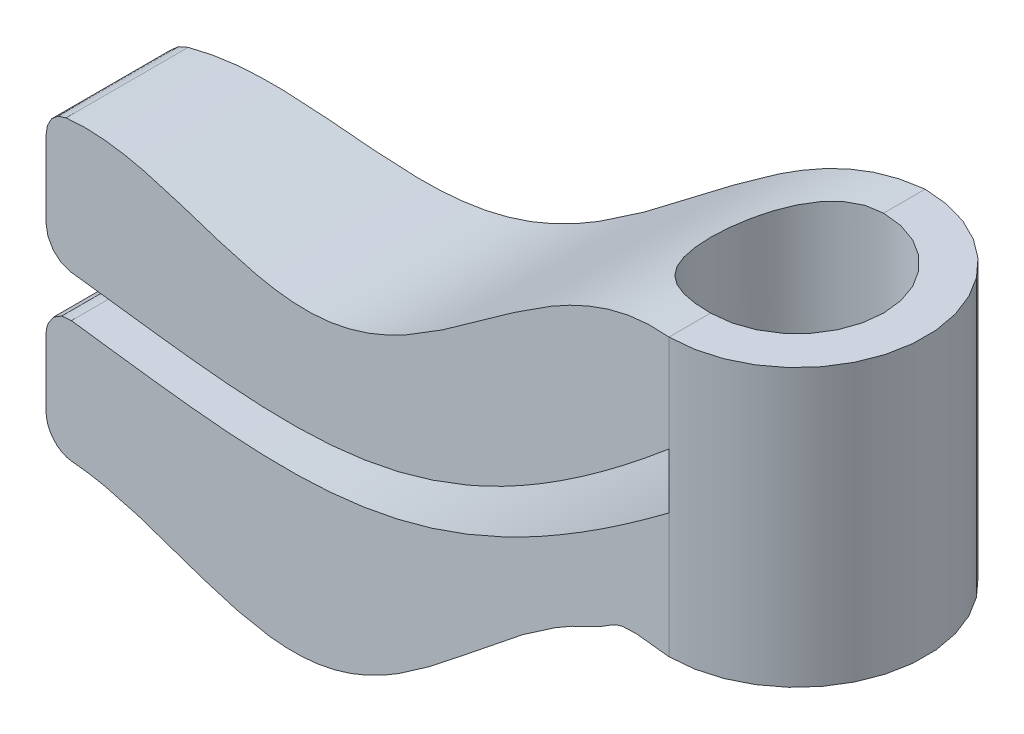
# Autodesk Inventor part: Fahne
Saved by Autodesk Inventor 2020 (Build 240168000, 168)
## iProperties
Created: 2020-05-10
Part Number: Fahne
Material: Generisch
Document SubType Name: Modeling
Designer: MartinDJay
Density: 1 g/cm^3
Appearance: Vorgabe
Author: MartinDJay
Autodesk Inventor part; units mm, degrees
ref_plane "YZ Plane" through (0, 0, 0) normal (1, 0, 0) x (0, 1, 0)
ref_plane "XZ Plane" through (0, 0, 0) normal (0, 1, 0) x (-1, 0, 0)
ref_plane "XY Plane" through (0, 0, 0) normal (0, 0, 1) x (1, 0, 0)
sketch "Skizze1" plane through (0, 0, 0) normal (0, 1, 0) x (-1, 0, 0)
  circle A0 centre (0, 0) radius 6.25
  circle A1 centre (0, 0) radius 9.25
  dimension "d0" = 12.5
  dimension "d2" = 3
  constraints: 2 centre point, 2 coincident
  measures "d0" diameter of A0
  measures "d2" radial gap between concentric circles of A1 A0
extrude "Extrusion1" add sketch "Skizze1" along normal blind 20
sketch "Skizze2" plane through (0, 20, 0) normal (0, 1, 0) x (1, 0, 0)
  circle A0 centre (0, 0) radius 9.25 projected
  line L0 (0, -9.25) -> (-50, -9.25)
  line L1 (-50, -9.25) -> (-50, 9.25)
  line L2 (-50, 9.25) -> (0, 9.25)
  line L3 (-50, 0) -> (0, 0) construction
  dimension "d5" = 50
  constraints: 8 end point, 2 horizontal, 2 point on circle, 2 tangent, 1 midpoint, 1 perpendicular, 1 point on line
  measures "d5" distance of L0.start L0.end
extrude "Extrusion2" add sketch "Skizze2" against normal blind 45 contours A0 L0 L1 L2
sketch "Skizze3" plane through (-50, 20, 9.25) normal (0, 0, 1) x (1, 0, 0)
  line L0 (0, 0) -> (0, -45) projected
  spline S0 degree 4 poles (50, -20) (33.6893, -20) (25.205, -49.5147) (14.9206, -32.0469) (0, -34.3156) knots 0 0 0 0 0 1 1 1 1 1
  line L1 (50, -20) -> (50, -45)
  line L2 (50, -45) -> (0, -45)
  line L3 (0, -45) -> (0, -34.3156)
  line L4 (59.25, -20) -> (50, -20) projected
  line L5 (50, -45) -> (0, -45) projected
  line L6 (50, -20) -> (50, 0) projected
  spline S1 degree 4 poles (50, 0) (34.1322, 0) (24.5091, -28.0895) (15.116, -8.5647) (0, -13.3156) knots 0 0 0 0 0 1 1 1 1 1
  line L7 (0, -13.3156) -> (0, 0)
  line L8 (0, 0) -> (50, 0) projected
  line L9 (59.25, 0) -> (50, 0) projected
  spline S2 degree 3 poles (50, -7) (29.5788, -24.5812) (20.0225, -22.4161) (0, -22.3156) knots 0 0 0 0 1 1 1 1
  spline S3 degree 3 poles (50, -11) (29.3142, -27.0201) (20.0053, -25.6187) (0, -25.3156) knots 0 0 0 0 1 1 1 1
  line L10 (0, -22.3156) -> (0, -25.3156)
  line L11 (50, -7) -> (50, -11)
  point P0 (30, -31.7804)
  point P1 (17, -36.3156)
  point P2 (30, -10.7804)
  point P3 (17, -14.3156)
  point P4 (30, -19.7804)
  point P5 (17, -22.3156)
  point P6 (30, -22.7804)
  point P7 (17, -25.3156)
  point P8 (0, -25.3156)
  dimension "d11" = 20
  dimension "d12" = 13
  dimension "d16" = 8
  dimension "d17" = 9
  dimension "d18" = 7
  dimension "d19" = 9
  dimension "d20" = 4
  dimension "d21" = 9
  dimension "d22" = 11
  dimension "d23" = 9
  dimension "d26" = 3
  dimension "d27" = 3
  dimension "d28" = 3
  constraints: 12 end point, 7 vertical alignment, 5 point on line, 2 horizontal, 2 perpendicular, 2 vertical, 1 collinear, 1 parallel, 16 other
  measures "d11" distance from line of L1 point (30, -31.78)
  measures "d12" horizontal distance of point (30, -31.78) point (17, -36.316)
  measures "d16" distance of point (17, -14.316) point (17, -22.316)
  measures "d17" distance of point (30, -10.78) point (30, -19.78)
  measures "d18" distance of L6.end L11.start
  measures "d19" distance of L7.start L10.start
  measures "d20" distance of L11.start L11.end
  measures "d21" distance of point (30, -22.78) point (30, -31.78)
  measures "d22" distance of point (17, -36.316) point (17, -25.316)
  measures "d23" distance of L3.end L10.end
  measures "d26" distance of point (30, -22.78) point (30, -19.78)
  measures "d27" distance of point (17, -22.316) point (17, -25.316)
  measures "d28" distance of L10.start L10.end
extrude "Extrusion3" cut sketch "Skizze3" against normal through all contours L8 S1 L0 | S2 L6 S3 L0 | S0 L1 L2 L0
sketch "Skizze4" plane through (0, 20, 0) normal (0, 1, 0) x (1, 0, 0)
  line L0 (-50, -9.25) -> (-50, 9.25) projected
  line L1 (-50, -9.25) -> (0, -9.25)
  line L2 (0, -9.25) -> (-50, -4.25)
  line L3 (-50, -4.25) -> (-50, -9.25)
  line L4 (-50, 0) -> (0, 0) construction
  line L5 (-50, 9.25) -> (0, 9.25)
  line L6 (0, 9.25) -> (-50, 4.25)
  line L7 (-50, 4.25) -> (-50, 9.25)
  dimension "d29" = 5
  constraints: 14 end point, 2 horizontal, 2 symmetric about line, 1 collinear, 1 midpoint, 1 point on line
  measures "d29" distance of L2.end L0.start
extrude "Extrusion4" cut sketch "Skizze4" against normal blind 45
fillet "Rundung1" radius 2 4 edges at (-50, 6.6844, 0) (-50, -2.3156, 0) (-50, -5.3156, 0) (-50, -14.3156, 0)
fillet "Rundung2" radius 2 1 edges at (-9.25, -3.2808, -0.0002)
fillet "Rundung3" radius 2 3 edges at (-9.25, 0, 0) (-5.0887, 0, 7.8545) (-5.0887, 0, -7.8545)
